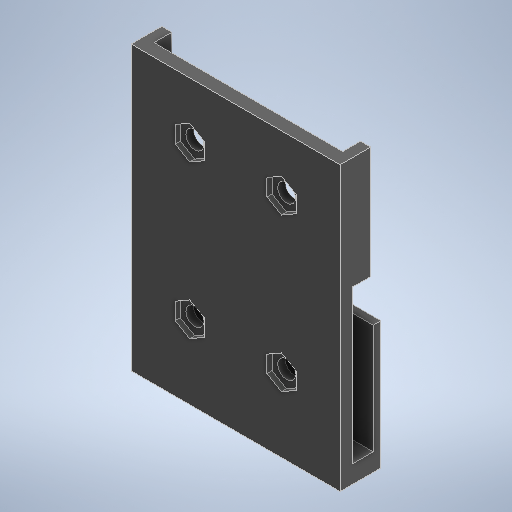
# Autodesk Inventor part: belt_end
Saved by Autodesk Inventor 2026.1 (Build 301233020, 233B)
## iProperties
Created: 2026-02-05
Part Number: belt_end
Material: 一般
Document SubType Name: Modeling
Designer: hibik
Density: 1 g/cm^3
Appearance: 既定
Author: hibik
Autodesk Inventor part; units mm, degrees
ref_plane "YZ Plane" through (0, 0, 0) normal (1, 0, 0) x (0, 1, 0)
ref_plane "XZ Plane" through (0, 0, 0) normal (0, 1, 0) x (-1, 0, 0)
ref_plane "XY Plane" through (0, 0, 0) normal (0, 0, 1) x (1, 0, 0)
sketch "スケッチ1" plane through (0, 0, 0) normal (0, 0, 1) x (1, 0, 0)
  line L0 (-20.5, 0) -> (20.5, 0)
  line L1 (20.5, 0) -> (20.5, 22)
  line L2 (20.5, 22) -> (-20.5, 22)
  line L3 (-20.5, 22) -> (-20.5, 0)
  point P0 (0, 0)
  point P1 (0, 0)
  dimension "d0" = 41
  dimension "d1" = 22
  constraints: 8 end point, 2 parallel, 1 coincident, 1 horizontal, 1 midpoint, 1 perpendicular
  measures "d0" distance of L2.end L1.end
  measures "d1" distance of L2.end L0.start
extrude "押し出し1" add sketch "スケッチ1" along normal blind 6
sketch "スケッチ2" plane through (0, 0, 0) normal (0, 0, -1) x (-1, 0, 0)
  line L0 (-18.5, 22) -> (18.5, 22)
  line L1 (18.5, 22) -> (18.5, 0)
  line L2 (18.5, 0) -> (-18.5, 0)
  line L3 (-18.5, 0) -> (-18.5, 22)
  line L4 (-20.5, 0) -> (-20.5, 22) projected
  line L5 (-20.5, 22) -> (20.5, 22) projected
  point P0 (0, 0)
  point P1 (0, 22)
  dimension "d4" = 2
  constraints: 8 end point, 2 midpoint, 2 parallel, 1 horizontal, 1 perpendicular
  measures "d4" distance between parallel lines of L4 L3
extrude "押し出し2" cut sketch "スケッチ2" against normal blind 3.5
sketch "スケッチ3" plane through (0, 0, 3.5) normal (0, 0, -1) x (-1, 0, 0)
  circle A0 centre (-9, 11) radius 1.75
  circle A1 centre (9, 11) radius 1.75
  line L0 (0, -4.4) -> (0, 26.4) projected
  line L1 (-18.5, 0) -> (-18.5, 22) projected
  point P0 (0, 0)
  point P1 (-18.5, 11)
  dimension "d7" = 3.5
  dimension "d8" = 18
  constraints: 2 centre point, 1 horizontal alignment, 1 midpoint, 1 other
  measures "d7" diameter of A0
  measures "d8" distance of A1.centre A0.centre
extrude "押し出し3" cut sketch "スケッチ3" along normal mid plane 50
sketch "スケッチ4" plane through (0, 0, 6) normal (0, 0, 1) x (1, 0, 0)
  circle A0 centre (-9, 11) radius 1.75 projected
  circle A1 centre (9, 11) radius 1.75 projected
  line L0 (-9, 7.7091) -> (-11.85, 9.3546)
  line L1 (-11.85, 9.3546) -> (-11.85, 12.6454)
  line L2 (-11.85, 12.6454) -> (-9, 14.2909)
  line L3 (-9, 14.2909) -> (-6.15, 12.6454)
  line L4 (-6.15, 12.6454) -> (-6.15, 9.3546)
  line L5 (-6.15, 9.3546) -> (-9, 7.7091)
  line L6 (9, 7.7091) -> (6.15, 9.3546)
  line L7 (6.15, 9.3546) -> (6.15, 12.6454)
  line L8 (6.15, 12.6454) -> (9, 14.2909)
  line L9 (9, 14.2909) -> (11.85, 12.6454)
  line L10 (11.85, 12.6454) -> (11.85, 9.3546)
  line L11 (11.85, 9.3546) -> (9, 7.7091)
  point P0 (0, 0)
  dimension "d11" = 5.7
  constraints: 24 end point, 2 coincident, 2 vertical, 1 parallel, 26 other
  measures "d11" distance between parallel lines of L1 L4
extrude "押し出し4" cut sketch "スケッチ4" against normal blind 1 contours A0 | A1 | L0 L1 L2 L3 L4 L5 | L6 L7 L8 L9 L10 L11
sketch "スケッチ5" plane through (-20.5, 0, 6) normal (0, -1, 0) x (1, 0, 0)
  line L0 (41, -2.5) -> (0, -2.5)
  line L1 (0, -2.5) -> (0, 0)
  line L2 (0, 0) -> (41, 0)
  line L3 (41, 0) -> (41, -2.5)
  line L4 (41, -6) -> (41, 0) projected
  line L5 (2, -2.5) -> (39, -2.5) projected
  point P0 (20.5, -6)
  constraints: 8 end point, 2 parallel, 2 point on line, 1 coincident, 1 horizontal, 1 perpendicular
extrude "押し出し5" add sketch "スケッチ5" along normal blind 33.5
sketch "スケッチ6" plane through (0, 0, 3.5) normal (0, 0, -1) x (-1, 0, 0)
  line L0 (-20.5, 22) -> (-20.5, -33.5) projected
  line L1 (-20.5, -33.5) -> (20.5, -33.5)
  line L2 (20.5, -33.5) -> (20.5, -30)
  line L3 (20.5, -30) -> (-20.5, -30)
  line L4 (-20.5, -30) -> (-20.5, -33.5)
  line L5 (20.5, 0) -> (20.5, -33.5) projected
  point P0 (0, 0)
  point P1 (-20.5, -30)
  dimension "d16" = 3.5
  constraints: 8 end point, 2 parallel, 1 horizontal, 1 perpendicular, 1 point on line
  measures "d16" distance of L1.end L2.end
extrude "押し出し6" add sketch "スケッチ6" along normal blind 4
sketch "スケッチ7" plane through (0, 0, -0.5) normal (0, 0, -1) x (-1, 0, 0)
  line L0 (-20.5, -33.5) -> (20.5, -33.5) projected
  line L1 (-20.5, -33.5) -> (20.5, -33.5)
  line L2 (20.5, -33.5) -> (20.5, -8.5)
  line L3 (20.5, -8.5) -> (-20.5, -8.5)
  line L4 (-20.5, -8.5) -> (-20.5, -33.5)
  point P0 (0, 0)
  dimension "d19" = 25
  constraints: 8 end point, 2 parallel, 1 horizontal, 1 perpendicular, 1 point on line
  measures "d19" distance of L3.end L0.start
extrude "押し出し7" add sketch "スケッチ7" along normal blind 1.5
pattern_linear "矩形状パターン1" count 2 spacing 30 along (0, -1, 0) of "押し出し4", "押し出し3"
